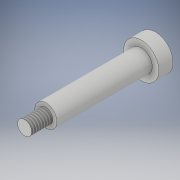
# Autodesk Inventor part: Tornillo_1
Saved by Autodesk Inventor 2019 (Build 230136000, 136)
## iProperties
Created: 2019-05-14
Part Number: Tornillo_1
Material: Generic
Document SubType Name: Modeling
Designer: Gustavo Marin
Density: 1 g/cm^3
Appearance: Default
Author: Gustavo Marin
Autodesk Inventor part; units mm, degrees
ref_plane "YZ Plane" through (0, 0, 0) normal (1, 0, 0) x (0, 1, 0)
ref_plane "XZ Plane" through (0, 0, 0) normal (0, 1, 0) x (-1, 0, 0)
ref_plane "XY Plane" through (0, 0, 0) normal (0, 0, 1) x (1, 0, 0)
sketch "Sketch1" plane through (0, 0, 0) normal (0, 1, 0) x (-1, 0, 0)
  line L0 (0, 0) -> (5.08, 0)
  line L1 (5.08, 0) -> (5.08, -15.24)
  line L2 (5.08, -15.24) -> (7.9375, -15.24)
  line L3 (7.9375, -15.24) -> (7.9375, -83.82)
  line L4 (7.9375, -83.82) -> (12.7, -83.82)
  line L5 (12.7, -83.82) -> (12.7, -93.98)
  line L6 (12.7, -93.98) -> (0, -93.98)
  line L7 (0, -93.98) -> (0, 0)
  dimension "d0" = 93.98
  dimension "d1" = 10.16
  dimension "d2" = 68.58
  dimension "d3" = 5.08
  dimension "d4" = 7.9375
  dimension "d5" = 12.7
  constraints: 16 end point, 7 perpendicular, 1 horizontal
  measures "d0" distance of L6.end L0.start
  measures "d1" distance between parallel lines of L6 L4
  measures "d2" distance between parallel lines of L2 L4
  measures "d3" distance between parallel lines of L1 L7
  measures "d4" distance between parallel lines of L7 L3
  measures "d5" distance between parallel lines of L7 L5
revolve "Revolution1" add sketch "Sketch1" angle 360 about axis through (0, 0, -93.98) along (0, 0, 1)
thread "Thread1" size "1/2-13 UNC" class "1A" standard "ANSI Unified Screw Threads" full length
body "Solid1"
